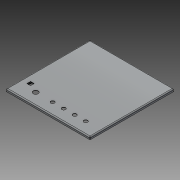
# Autodesk Inventor part: AE 1050_01_00 Tuer
Saved by Autodesk Inventor 2016 (Build 200138000, 138)
## iProperties
Category: PARTsolutions
Company: RITTAL
Created: 2014-04-04
Part Number: AE 1050_01_00 Tuer
Catalog Web Link: www.cadenas.de
Description: Einzeltür AE-Einzeltür AE
Vendor: RITTAL
Document SubType Name: Modeling
Designer: PARTuser1
Manufacturer: RITTAL
Density: 1 g/cm^3
Material: Generic
Appearance: RGB(195.00000357627781,201.00000321865156,196.00000351667384)
PSOL_IDENT_0: {$CADENAS_DATA\23d-libs\rittal\schaltschranksys\kompakt_schaltschr\ae\parts_ae\einzeltuer_ae.prj},18
PSOL_IDENT_1: 3 {VTYP=3D},{NB=1050_01_01 (1)},{LINA=1050_01_01 (1)},{NN=Einzeltür AE},{DATE=25.09.2013 06:56:31},{
PSOL_IDENT_2: GEOMDATE=25.09.2013 08:56:00},{VERSION=},{LINEID=180},{LINESUBID=-1},{WBVAR=DETAIL}  {NB=1050_01_01
PSOL_IDENT_3: (1)},{LINA=1050_01_01 (1)},{KT=DUMMY},{BEST=1050},{VERS=1},{DETAIL=1},{A=500.000},{B=500.000},{C=210
PSOL_IDENT_4: .000},{D=303.000},{E=113.000},{F=38.000},{G=30.000},{H=445.000},{I=355.000},{J=1.750},{K=470.000},{P
PSOL_IDENT_5: =410.000},{Q=449.000},{R=495.000},{S=495.000},{T=356.300},{U=425.000},{V=17.000},{W=438.000},{X=411.
PSOL_IDENT_6: 000},{Y=423.000},{B1=500},{H1=500},{T1=210},{F1=449},{G1=470},{S1=2.5},{GEW=16.8},{XX=1.550}
CNS_NN: Einzeltür AE
CNS_NT: Einzeltür AE
CNS_NB: 1050_01_01 (1)
CNS_NBSYN: $BEST._01_01 ($DETAIL.)
CNS_LINA: 1050_01_01 (1)
CNS_BEST: 1050
CNS_VERS: 1
CNS_DETAIL: 1
CNS_A: 500.000
CNS_B: 500.000
CNS_C: 210.000
CNS_D: 303.000
CNS_E: 113.000
CNS_F: 38.000
CNS_G: 30.000
CNS_H: 445.000
CNS_I: 355.000
CNS_J: 1.750
CNS_K: 470.000
CNS_P: 410.000
CNS_Q: 449.000
CNS_R: 495.000
CNS_S: 495.000
CNS_T: 356.300
CNS_U: 425.000
CNS_V: 17.000
CNS_W: 438.000
CNS_X: 411.000
CNS_Y: 423.000
CNS_B1: 500
CNS_H1: 500
CNS_T1: 210
CNS_F1: 449
CNS_G1: 470
CNS_S1: 2.5
CNS_GEW: 16.8
CNS_XX: 1.550
SUPPLIER: RITTAL
ARTICLENO: 1050_01_01 (1)
BOMINFO: 1050_01_01 (1)
CREATOR: CADENAS GmbH
Title: 1050_01_01 (1)
Author: Cadenas PARTsolutions
Comments: Einzeltür AE
Autodesk Inventor part; units mm, degrees
sketch "Skizze_6" plane through (0, 0, 0) normal (1, 0, 0) x (0, 0, -1)
  line L0 (0, 242) -> (0, -242)
  arc A0 (0, -242) -> (5.5, -247.5) centre (5.5, -242) ccw
  line L1 (5.5, -247.5) -> (15, -247.5)
  line L2 (15, -247.5) -> (15, -245.75)
  line L3 (15, -245.75) -> (5.5, -245.75)
  arc A1 (1.75, -242) -> (5.5, -245.75) centre (5.5, -242) ccw
  line L4 (1.75, -242) -> (1.75, 242)
  arc A2 (5.5, 245.75) -> (1.75, 242) centre (5.5, 242) ccw
  line L5 (5.5, 245.75) -> (15, 245.75)
  line L6 (15, 245.75) -> (15, 247.5)
  line L7 (15, 247.5) -> (5.5, 247.5)
  arc A3 (5.5, 247.5) -> (0, 242) centre (5.5, 242) ccw
  constraints: 16 end point, 8 point on circle, 4 centre point
extrude "Extrusion1" add sketch "Skizze_6" along normal mid plane 484
sketch "Skizze_7" plane through (242, 0, 0) normal (1, 0, 0) x (0, 0, -1)
  line L0 (0, -242) -> (1.75, -242)
  arc A0 (1.75, -242) -> (5.5, -245.75) centre (5.5, -242) ccw
  line L1 (5.5, -245.75) -> (15, -245.75)
  line L2 (15, -245.75) -> (15, -247.5)
  line L3 (15, -247.5) -> (5.5, -247.5)
  arc A1 (0, -242) -> (5.5, -247.5) centre (5.5, -242) ccw
  line L4 (0, -242) -> (1.75, -242)
  constraints: 10 end point, 4 point on circle, 2 centre point
sketch "Skizze_8" plane through (242, 0, 0) normal (1, 0, 0) x (0, 0, -1)
  line L0 (1.75, 242) -> (0, 242)
  arc A0 (5.5, 247.5) -> (0, 242) centre (5.5, 242) ccw
  line L1 (5.5, 247.5) -> (15, 247.5)
  line L2 (15, 247.5) -> (15, 245.75)
  line L3 (15, 245.75) -> (5.5, 245.75)
  arc A1 (5.5, 245.75) -> (1.75, 242) centre (5.5, 242) ccw
  line L4 (1.75, 242) -> (0, 242)
  constraints: 10 end point, 4 point on circle, 2 centre point
sketch "Skizze_9" plane through (-242, 0, 0) normal (1, 0, 0) x (0, 0, -1)
  line L0 (0, -242) -> (1.75, -242)
  arc A0 (1.75, -242) -> (5.5, -245.75) centre (5.5, -242) ccw
  line L1 (5.5, -245.75) -> (15, -245.75)
  line L2 (15, -245.75) -> (15, -247.5)
  line L3 (15, -247.5) -> (5.5, -247.5)
  arc A1 (0, -242) -> (5.5, -247.5) centre (5.5, -242) ccw
  line L4 (0, -242) -> (1.75, -242)
  constraints: 10 end point, 4 point on circle, 2 centre point
sketch "Skizze_10" plane through (-242, 0, 0) normal (1, 0, 0) x (0, 0, -1)
  line L0 (1.75, 242) -> (0, 242)
  arc A0 (5.5, 247.5) -> (0, 242) centre (5.5, 242) ccw
  line L1 (5.5, 247.5) -> (15, 247.5)
  line L2 (15, 247.5) -> (15, 245.75)
  line L3 (15, 245.75) -> (5.5, 245.75)
  arc A1 (5.5, 245.75) -> (1.75, 242) centre (5.5, 242) ccw
  line L4 (1.75, 242) -> (0, 242)
  constraints: 10 end point, 4 point on circle, 2 centre point
sketch "Skizze_11" plane through (0, 0, 0) normal (0, 1, 0) x (1, 0, 0)
  line L0 (242, 1.75) -> (242, 0)
  arc A0 (242, 0) -> (247.5, 5.5) centre (242, 5.5) ccw
  line L1 (247.5, 5.5) -> (247.5, 15)
  line L2 (247.5, 15) -> (245.75, 15)
  line L3 (245.75, 15) -> (245.75, 5.5)
  arc A1 (242, 1.75) -> (245.75, 5.5) centre (242, 5.5) ccw
  constraints: 8 end point, 4 point on circle, 2 centre point
sketch "Skizze_12" plane through (0, 0, 0) normal (0, 1, 0) x (1, 0, 0)
  line L0 (-247.5, 15) -> (-247.5, 5.5)
  arc A0 (-247.5, 5.5) -> (-242, 0) centre (-242, 5.5) ccw
  line L1 (-242, 0) -> (-242, 1.75)
  arc A1 (-245.75, 5.5) -> (-242, 1.75) centre (-242, 5.5) ccw
  line L2 (-245.75, 5.5) -> (-245.75, 15)
  line L3 (-245.75, 15) -> (-247.5, 15)
  constraints: 8 end point, 4 point on circle, 2 centre point
sketch "Skizze_13" plane through (0, 0, 0) normal (0, 1, 0) x (1, 0, 0)
  line L0 (229.8, 1.75) -> (241.7, 1.75)
  line L1 (241.7, 1.75) -> (241.7, 2.8035)
  arc A0 (241.7, 2.8035) -> (229.8, 2.8035) centre (235.75, 2.2767) ccw
  line L2 (229.8, 2.8035) -> (229.8, 1.75)
  constraints: 6 end point, 2 point on circle, 1 centre point
extrude "Extrusion2" add sketch "Skizze_13" along normal mid plane 471.5
sketch "Skizze_14" plane through (0, 0, 0) normal (0, 1, 0) x (1, 0, 0)
  line L0 (-241.7, 1.75) -> (-229.8, 1.75)
  line L1 (-229.8, 1.75) -> (-229.8, 2.8035)
  arc A0 (-229.8, 2.8035) -> (-241.7, 2.8035) centre (-235.75, 2.2767) ccw
  line L2 (-241.7, 2.8035) -> (-241.7, 1.75)
  constraints: 6 end point, 2 point on circle, 1 centre point
extrude "Extrusion3" add sketch "Skizze_14" along normal mid plane 471.5
sketch "Skizze_19" plane through (0, 0, 0) normal (1, 0, 0) x (0, 0, -1)
  line L0 (1.75, -241.7) -> (2.8035, -241.7)
  arc A0 (2.8035, -241.7) -> (2.8035, -229.8) centre (2.2767, -235.75) ccw
  line L1 (2.8035, -229.8) -> (1.75, -229.8)
  line L2 (1.75, -229.8) -> (1.75, -241.7)
  constraints: 6 end point, 2 point on circle, 1 centre point
extrude "Extrusion4" add sketch "Skizze_19" along normal mid plane 483.4
sketch "Skizze_20" plane through (0, 0, 0) normal (1, 0, 0) x (0, 0, -1)
  line L0 (1.75, 229.8) -> (2.8035, 229.8)
  arc A0 (2.8035, 229.8) -> (2.8035, 241.7) centre (2.2767, 235.75) ccw
  line L1 (2.8035, 241.7) -> (1.75, 241.7)
  line L2 (1.75, 241.7) -> (1.75, 229.8)
  constraints: 6 end point, 2 point on circle, 1 centre point
extrude "Extrusion5" add sketch "Skizze_20" along normal mid plane 483.4
sketch "Skizze_15" plane through (0, 0, 0) normal (0, 1, 0) x (1, 0, 0)
  line L0 (-246.7, 1.75) -> (-241.7, 1.75)
  line L1 (-241.7, 1.75) -> (-241.7, 2.8035)
  arc A0 (-235.75, 8.25) -> (-241.7, 2.8035) centre (-235.75, 2.2767) ccw
  line L2 (-235.75, 8.25) -> (235.75, 8.25)
  arc A1 (241.7, 2.8035) -> (235.75, 8.25) centre (235.75, 2.2767) ccw
  line L3 (241.7, 2.8035) -> (241.7, 1.75)
  line L4 (241.7, 1.75) -> (246.7, 1.75)
  line L5 (246.7, 1.75) -> (246.7, 13.25)
  line L6 (246.7, 13.25) -> (-246.7, 13.25)
  line L7 (-246.7, 13.25) -> (-246.7, 1.75)
  constraints: 16 end point, 4 point on circle, 2 centre point
extrude "Extrusion6" cut sketch "Skizze_15" along normal mid plane 483.5
extrude "Extrusion7" add sketch "Skizze_11" along normal mid plane 484
extrude "Extrusion8" add sketch "Skizze_12" along normal mid plane 484
revolve "Revolution1" add sketch "Skizze_7" angle 90 about axis through (242, -242, 0) along (0, 0, 1)
revolve "Revolution2" add sketch "Skizze_9" angle 90 about axis through (-242, -242, 0) along (0, 0, -1)
revolve "Revolution3" add sketch "Skizze_10" angle 90 about axis through (-242, 242, -1.75) along (0, 0, 1)
revolve "Revolution4" add sketch "Skizze_8" angle 90 about axis through (242, 242, -1.75) along (0, 0, -1)
sketch "Skizze_4" plane through (0, 0, 0) normal (0, 1, 0) x (1, 0, 0)
  line L0 (205.5, 15.75) -> (205.5, 14.75)
  line L1 (205.5, 14.75) -> (216.595, 14.75)
  arc A0 (217.59, 13.8495) -> (216.595, 14.75) centre (216.595, 13.75) ccw
  line L2 (217.59, 13.8495) -> (218.6199, 3.551)
  arc A1 (218.6199, 3.551) -> (220.61, 1.75) centre (220.61, 3.75) ccw
  line L3 (220.61, 1.75) -> (230.5, 1.75)
  line L4 (230.5, 1.75) -> (230.5, 2.75)
  line L5 (230.5, 2.75) -> (220.61, 2.75)
  arc A2 (219.6149, 3.6505) -> (220.61, 2.75) centre (220.61, 3.75) ccw
  line L6 (219.6149, 3.6505) -> (218.5851, 13.949)
  arc A3 (218.5851, 13.949) -> (216.595, 15.75) centre (216.595, 13.75) ccw
  line L7 (216.595, 15.75) -> (205.5, 15.75)
  constraints: 16 end point, 8 point on circle, 4 centre point
extrude "Extrusion9" add sketch "Skizze_4" along normal mid plane 438
sketch "Skizze_5" plane through (0, 0, 0) normal (0, 1, 0) x (1, 0, 0)
  line L0 (-230.5, 2.75) -> (-230.5, 1.75)
  line L1 (-230.5, 1.75) -> (-220.61, 1.75)
  arc A0 (-220.61, 1.75) -> (-218.6199, 3.551) centre (-220.61, 3.75) ccw
  line L2 (-218.6199, 3.551) -> (-217.59, 13.8495)
  arc A1 (-216.595, 14.75) -> (-217.59, 13.8495) centre (-216.595, 13.75) ccw
  line L3 (-216.595, 14.75) -> (-205.5, 14.75)
  line L4 (-205.5, 14.75) -> (-205.5, 15.75)
  line L5 (-205.5, 15.75) -> (-216.595, 15.75)
  arc A2 (-216.595, 15.75) -> (-218.5851, 13.949) centre (-216.595, 13.75) ccw
  line L6 (-218.5851, 13.949) -> (-219.6149, 3.6505)
  arc A3 (-220.61, 2.75) -> (-219.6149, 3.6505) centre (-220.61, 3.75) ccw
  line L7 (-220.61, 2.75) -> (-230.5, 2.75)
  constraints: 16 end point, 8 point on circle, 4 centre point
extrude "Extrusion10" add sketch "Skizze_5" along normal mid plane 438
sketch "Skizze_21" plane through (0, -190.6, 0) normal (0, 1, 0) x (1, 0, 0)
  arc A0 (242.4, 12.35) -> (242.4, 4.05) centre (242.4, 8.2) ccw
  line L0 (242.4, 4.05) -> (246.35, 4.05)
  line L1 (246.35, 4.05) -> (246.35, 5.5)
  line L2 (246.35, 5.5) -> (242.4, 5.5)
  arc A1 (242.4, 10.9) -> (242.4, 5.5) centre (242.4, 8.2) ccw
  line L3 (242.4, 10.9) -> (246.35, 10.9)
  line L4 (246.35, 10.9) -> (246.35, 12.35)
  line L5 (246.35, 12.35) -> (242.4, 12.35)
  constraints: 12 end point, 4 point on circle, 2 centre point
extrude "Extrusion11" add sketch "Skizze_21" along normal mid plane 26
sketch "Skizze_22" plane through (0, 190.6, 0) normal (0, 1, 0) x (1, 0, 0)
  arc A0 (242.4, 12.35) -> (242.4, 4.05) centre (242.4, 8.2) ccw
  line L0 (242.4, 4.05) -> (246.35, 4.05)
  line L1 (246.35, 4.05) -> (246.35, 5.5)
  line L2 (246.35, 5.5) -> (242.4, 5.5)
  arc A1 (242.4, 10.9) -> (242.4, 5.5) centre (242.4, 8.2) ccw
  line L3 (242.4, 10.9) -> (246.35, 10.9)
  line L4 (246.35, 10.9) -> (246.35, 12.35)
  line L5 (246.35, 12.35) -> (242.4, 12.35)
  constraints: 12 end point, 4 point on circle, 2 centre point
extrude "Extrusion12" add sketch "Skizze_22" along normal mid plane 26
sketch "Skizze_24" plane through (0, 0, 0) normal (0, 0, 1) x (1, 0, 0)
  line L0 (-211.05, -161.05) -> (-188.95, -161.05)
  line L1 (-188.95, -161.05) -> (-188.95, -138.95)
  line L2 (-188.95, -138.95) -> (-211.05, -138.95)
  line L3 (-211.05, -138.95) -> (-211.05, -161.05)
  constraints: 8 end point
extrude "Extrusion13" cut sketch "Skizze_24" against normal blind 1.75
sketch "Skizze_41" plane through (0, 0, 0) normal (0, 0, 1) x (1, 0, 0)
  line L0 (-211.05, 138.95) -> (-188.95, 138.95)
  line L1 (-188.95, 138.95) -> (-188.95, 161.05)
  line L2 (-188.95, 161.05) -> (-211.05, 161.05)
  line L3 (-211.05, 161.05) -> (-211.05, 138.95)
  constraints: 8 end point
extrude "Extrusion14" [suppressed]
sketch "Sketch19" plane through (216.595, 219, -15.75) normal (0, 0, -1) x (-1, 0, 0)
  point P0 (5.095, -406.5)
hole "Drilling 1" at (211.5, -187.5, -15.75) direction (0, 0, 1) diameter 3.7 depth 1
pattern_linear "Rectangular Pattern1" count 16 spacing 25 along (0, 1, 0) of "Drilling 1"
sketch "Sketch20" plane through (-205.5, 219, -15.75) normal (0, 0, -1) x (-1, 0, 0)
  point P0 (6, -406.5)
hole "Drilling 2" at (-211.5, -187.5, -15.75) direction (0, 0, 1) diameter 3.7 depth 1
pattern_linear "Rectangular Pattern2" count 16 spacing 25 along (0, 1, 0) of "Drilling 2"
sketch "Skizze_31" plane through (0, 0, -15.75) normal (0, 0, 1) x (1, 0, 0)
  line L0 (-215.8, 162.5147) -> (-215.8, 137.4853)
  arc A0 (-215.8, 137.4853) -> (-214.0426, 133.2426) centre (-209.8, 137.4853) ccw
  line L1 (-214.0426, 133.2426) -> (-207.2574, 126.4574)
  arc A1 (-205.5, 122.2147) -> (-207.2574, 126.4574) centre (-211.5, 122.2147) ccw
  line L2 (-205.5, 122.2147) -> (-205.5, -122.2147)
  arc A2 (-207.2574, -126.4574) -> (-205.5, -122.2147) centre (-211.5, -122.2147) ccw
  line L3 (-207.2574, -126.4574) -> (-214.0426, -133.2426)
  arc A3 (-214.0426, -133.2426) -> (-215.8, -137.4853) centre (-209.8, -137.4853) ccw
  line L4 (-215.8, -137.4853) -> (-215.8, -162.5147)
  arc A4 (-215.8, -162.5147) -> (-214.0426, -166.7574) centre (-209.8, -162.5147) ccw
  line L5 (-214.0426, -166.7574) -> (-207.2574, -173.5426)
  arc A5 (-205.5, -177.7853) -> (-207.2574, -173.5426) centre (-211.5, -177.7853) ccw
  line L6 (-205.5, -177.7853) -> (-205.5, -213)
  arc A6 (-211.5, -219) -> (-205.5, -213) centre (-211.5, -213) ccw
  line L7 (-211.5, -219) -> (-212.5, -219)
  line L8 (-212.5, -219) -> (-212.5, -224)
  line L9 (-212.5, -224) -> (212.5, -224)
  line L10 (212.5, -224) -> (212.5, -219)
  line L11 (212.5, -219) -> (211.5, -219)
  arc A7 (205.5, -213) -> (211.5, -219) centre (211.5, -213) ccw
  line L12 (205.5, -213) -> (205.5, -177.7853)
  arc A8 (207.2574, -173.5426) -> (205.5, -177.7853) centre (211.5, -177.7853) ccw
  line L13 (207.2574, -173.5426) -> (214.0426, -166.7574)
  arc A9 (214.0426, -166.7574) -> (215.8, -162.5147) centre (209.8, -162.5147) ccw
  line L14 (215.8, -162.5147) -> (215.8, -137.4853)
  arc A10 (215.8, -137.4853) -> (214.0426, -133.2426) centre (209.8, -137.4853) ccw
  line L15 (214.0426, -133.2426) -> (207.2574, -126.4574)
  arc A11 (205.5, -122.2147) -> (207.2574, -126.4574) centre (211.5, -122.2147) ccw
  line L16 (205.5, -122.2147) -> (205.5, 122.2147)
  arc A12 (207.2574, 126.4574) -> (205.5, 122.2147) centre (211.5, 122.2147) ccw
  line L17 (207.2574, 126.4574) -> (214.0426, 133.2426)
  arc A13 (214.0426, 133.2426) -> (215.8, 137.4853) centre (209.8, 137.4853) ccw
  line L18 (215.8, 137.4853) -> (215.8, 162.5147)
  arc A14 (215.8, 162.5147) -> (214.0426, 166.7574) centre (209.8, 162.5147) ccw
  line L19 (214.0426, 166.7574) -> (207.2574, 173.5426)
  arc A15 (205.5, 177.7853) -> (207.2574, 173.5426) centre (211.5, 177.7853) ccw
  line L20 (205.5, 177.7853) -> (205.5, 213)
  arc A16 (211.5, 219) -> (205.5, 213) centre (211.5, 213) ccw
  line L21 (211.5, 219) -> (212.5, 219)
  line L22 (212.5, 219) -> (212.5, 224)
  line L23 (212.5, 224) -> (-212.5, 224)
  line L24 (-212.5, 224) -> (-212.5, 219)
  line L25 (-212.5, 219) -> (-211.5, 219)
  arc A17 (-205.5, 213) -> (-211.5, 219) centre (-211.5, 213) ccw
  line L26 (-205.5, 213) -> (-205.5, 177.7853)
  arc A18 (-207.2574, 173.5426) -> (-205.5, 177.7853) centre (-211.5, 177.7853) ccw
  line L27 (-207.2574, 173.5426) -> (-214.0426, 166.7574)
  arc A19 (-214.0426, 166.7574) -> (-215.8, 162.5147) centre (-209.8, 162.5147) ccw
  constraints: 56 end point, 40 point on circle, 20 centre point
extrude "Extrusion15" cut sketch "Skizze_31" along normal blind 1
sketch "Sketch22" plane through (216.595, -219, -15.75) normal (0, 0, -1) x (-1, 0, 0)
  point P0 (5.095, 6.5)
hole "Drilling 3" at (211.5, -212.5, -15.75) direction (0, 0, 1) diameter 6.5 depth 1
sketch "Sketch23" plane through (216.595, -219, -15.75) normal (0, 0, -1) x (-1, 0, 0)
  point P0 (5.095, 431.5)
hole "Drilling 4" at (211.5, 212.5, -15.75) direction (0, 0, 1) diameter 6.5 depth 1
sketch "Sketch24" plane through (-216.595, -219, -15.75) normal (0, 0, -1) x (-1, 0, 0)
  point P0 (-5.095, 6.5)
hole "Drilling 5" at (-211.5, -212.5, -15.75) direction (0, 0, 1) diameter 6.5 depth 1
sketch "Sketch25" plane through (-216.595, -219, -15.75) normal (0, 0, -1) x (-1, 0, 0)
  point P0 (-5.095, 431.5)
hole "Drilling 6" at (-211.5, 212.5, -15.75) direction (0, 0, 1) diameter 6.5 depth 1
ref_plane "DPB21_XY" through (247.5, 247.5, 0) normal (0, 0, 1) x (1, 0, 0)
ref_plane "DPB21_YZ" through (247.5, 247.5, 0) normal (1, 0, 0) x (0, 1, 0)
ref_plane "DPB21_ZX" through (247.5, 247.5, 0) normal (0, 1, 0) x (0, 0, 1)
ref_plane "DPB211_XY" through (250, 247.5, 0) normal (0, 0, 1) x (1, 0, 0)
ref_plane "DPB211_YZ" through (250, 247.5, 0) normal (1, 0, 0) x (0, 1, 0)
ref_plane "DPB211_ZX" through (250, 247.5, 0) normal (0, 1, 0) x (0, 0, 1)
ref_plane "DPB22_XY" through (-247.5, 247.5, 0) normal (0, 0, 1) x (1, 0, 0)
ref_plane "DPB22_YZ" through (-247.5, 247.5, 0) normal (1, 0, 0) x (0, 1, 0)
ref_plane "DPB22_ZX" through (-247.5, 247.5, 0) normal (0, 1, 0) x (0, 0, 1)
ref_plane "DPB41_XY" through (205.5, -219, 0) normal (0, 0, 1) x (1, 0, 0)
ref_plane "DPB41_YZ" through (205.5, -219, 0) normal (1, 0, 0) x (0, 1, 0)
ref_plane "DPB41_ZX" through (205.5, -219, 0) normal (0, 1, 0) x (0, 0, 1)
ref_plane "DPB42_XY" through (-205.5, -219, 0) normal (0, 0, 1) x (1, 0, 0)
ref_plane "DPB42_YZ" through (-205.5, -219, 0) normal (1, 0, 0) x (0, 1, 0)
ref_plane "DPB42_ZX" through (-205.5, -219, 0) normal (0, 1, 0) x (0, 0, 1)
ref_plane "DPB51_XY" through (-211.5, -212.5, 0) normal (0, 0, 1) x (1, 0, 0)
ref_plane "DPB51_YZ" through (-211.5, -212.5, 0) normal (1, 0, 0) x (0, 1, 0)
ref_plane "DPB51_ZX" through (-211.5, -212.5, 0) normal (0, 1, 0) x (0, 0, 1)
ref_plane "DPB52_XY" through (211.5, -212.5, 0) normal (0, 0, 1) x (1, 0, 0)
ref_plane "DPB52_YZ" through (211.5, -212.5, 0) normal (1, 0, 0) x (0, 1, 0)
ref_plane "DPB52_ZX" through (211.5, -212.5, 0) normal (0, 1, 0) x (0, 0, 1)
ref_plane "tuer_XY" through (242.4, -190.6, -8.2) normal (0, 1, 0) x (1, 0, 0)
ref_plane "tuer_YZ" through (242.4, -190.6, -8.2) normal (1, 0, 0) x (0, 0, -1)
ref_plane "tuer_ZX" through (242.4, -190.6, -8.2) normal (0, 0, -1) x (0, 1, 0)
ref_plane "verschluss_XY" through (-200, -150, 0) normal (0, 0, 1) x (1, 0, 0)
ref_plane "verschluss_YZ" through (-200, -150, 0) normal (1, 0, 0) x (0, 1, 0)
ref_plane "verschluss_ZX" through (-200, -150, 0) normal (0, 1, 0) x (0, 0, 1)
ref_plane "verschluss2_XY" through (-200, 150, 0) normal (0, 0, 1) x (1, 0, 0)
ref_plane "verschluss2_YZ" through (-200, 150, 0) normal (1, 0, 0) x (0, 1, 0)
ref_plane "verschluss2_ZX" through (-200, 150, 0) normal (0, 1, 0) x (0, 0, 1)
sketch "Sketch26" plane through (-242, -242, 0) normal (0, 0, 1) x (1, 0, 0)
  line L0 (102, 62) -> (442, 62) construction
  circle A0 centre (397, 62) radius 11
  circle A1 centre (332, 62) radius 11
  circle A2 centre (267, 62) radius 11
  circle A3 centre (202, 62) radius 11
  circle A4 centre (102, 62) radius 15
  point P0 (242, 242)
  dimension "d88" = 340
  dimension "d90" = 22
  dimension "d91" = 22
  dimension "d92" = 22
  dimension "d93" = 22
  dimension "d95" = 30
  dimension "d96" = 65
  dimension "d97" = 65
  dimension "d98" = 65
  dimension "d99" = 100
  dimension "d110" = 180
  dimension "d111" = 140
  constraints: 5 centre point, 4 point on line, 2 coincident, 2 end point, 1 horizontal
  measures "d88" distance of L0.start L0.end
  measures "d90" diameter of A0
  measures "d91" diameter of A1
  measures "d92" diameter of A2
  measures "d93" diameter of A3
  measures "d95" diameter of A4
  measures "d96" distance of A1.centre point (397, 62)
  measures "d97" distance of A1.centre A2.centre
  measures "d98" distance of A2.centre A3.centre
  measures "d99" distance of A3.centre L0.start
  measures "d110" distance from line of L0 point (242, 242)
  measures "d111" horizontal distance of point (242, 242) L0.start
extrude "Extrusion16" cut sketch "Sketch26" against normal blind 10
sketch "Sketch27" plane through (0, 0, 0) normal (0, 0, 1) x (1, 0, 0)
  line L0 (-200, 210) -> (200, 210)
  line L1 (200, 210) -> (200, -90)
  line L2 (200, -90) -> (-200, -90)
  line L3 (-200, -90) -> (-200, 210)
  line L4 (-200, 210) -> (200, -90) construction
  line L5 (-200, -90) -> (200, 210) construction
  point P0 (0, 0)
  point P1 (0, -90)
  dimension "d107" = 400
  dimension "d108" = 300
  dimension "d109" = 90
  constraints: 12 end point, 2 parallel, 1 horizontal, 1 midpoint, 1 perpendicular, 1 vertical alignment
  measures "d107" distance of L1.end L2.end
  measures "d108" distance of L0.end L1.end
  measures "d109" distance from line of point (0, 0) L2
body "Solid1"
